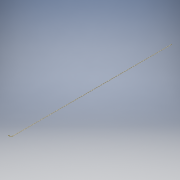
# Autodesk Inventor part: +XPanel_AntennaDeployed
Saved by Autodesk Inventor 2018 (Build 220112000, 112)
## iProperties
Created: 2018-11-03
Part Number: +XPanel_AntennaDeployed
Material: Titanium
Document SubType Name: Modeling
Designer: Bradley
Density: 4.51 g/cm^3
Appearance: Nickel
Author: Bradley
Autodesk Inventor part; units mm, degrees
ref_plane "YZ Plane" through (0, 0, 0) normal (1, 0, 0) x (0, 1, 0)
ref_plane "XZ Plane" through (0, 0, 0) normal (0, 1, 0) x (-1, 0, 0)
ref_plane "XY Plane" through (0, 0, 0) normal (0, 0, 1) x (1, 0, 0)
sketch "Sketch1" plane through (0, 0, 0) normal (0, 0, 1) x (1, 0, 0)
  line L0 (-3, -1.5) -> (-2, -1.5)
  line L1 (0, 0) -> (0, 167.5)
  spline S0 degree 4 poles (0, 0) (0, -0.375) (0, -1.125) (-0.9687, -1.5) (-1.6562, -1.5) (-2, -1.5) knots 0 0 0 0 0 0.5 1 1 1 1 1
  dimension "d0" = 1
  dimension "d1" = 2
  dimension "d2" = 1.5
  dimension "d18" = 169
  constraints: 5 end point, 2 horizontal, 2 vertical, 2 other
  measures "d0" distance of L0.start L0.end
  measures "d1" distance from line of L0.end L1
  measures "d2" distance from line of L1.start L0
  measures "d18" distance from line of L0 L1.end
sketch "Sketch3" plane through (0, 0, 0) normal (0, 1, 0) x (-1, 0, 0)
  circle A0 centre (0, 0) radius 0.25
  dimension "d7" = 0.5
  constraints: 1 centre point, 1 coincident
  measures "d7" diameter of A0
sweep "Sweep2" add profiles "Sketch3" path "Sketch1"
body "Solid2"
